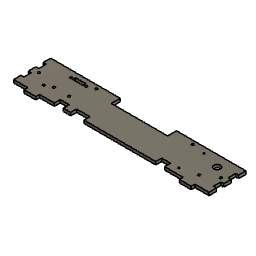
move_base_sidewall_1 (Autodesk Fusion 360 design; units mm, degrees)
Autodesk Fusion 360 part; units mm, degrees
note: some values were not read from the file. Set by a fixed rule: which sketch regions a step uses.
sketch "スケッチ1" plane through (0, 0, 0) normal (0, 1, 0) x (1, 0, 0)
  line L0 (-132, 0) -> (132, 0)
  line L1 (-132, 0) -> (-132, -10)
  line L2 (-132, -10) -> (-128, -10)
  line L3 (-128, -10) -> (-128, -20)
  line L4 (-128, -20) -> (-132, -20)
  line L5 (-132, -20) -> (-132, -30)
  line L6 (-132, -30) -> (-128, -30)
  line L7 (-128, -30) -> (-128, -40)
  line L8 (-128, -40) -> (-132, -40)
  line L9 (-132, -40) -> (-132, -50)
  line L10 (-132, -50) -> (-77, -50)
  line L11 (-77, -50) -> (-77, -42)
  line L12 (132, 0) -> (132, -10)
  line L13 (132, -10) -> (128, -10)
  line L14 (128, -10) -> (128, -20)
  line L15 (128, -20) -> (132, -20)
  line L16 (132, -20) -> (132, -30)
  line L17 (132, -30) -> (128, -30)
  line L18 (128, -30) -> (128, -40)
  line L19 (128, -40) -> (132, -40)
  line L20 (132, -40) -> (132, -50)
  line L21 (132, -50) -> (72, -50)
  line L22 (72, -50) -> (72, -42)
  line L23 (-77, -42) -> (-65, -42)
  line L24 (-65, -42) -> (-65, -50)
  line L25 (-37, -50) -> (60, -50)
  line L26 (60, -50) -> (60, -42)
  line L27 (60, -42) -> (72, -42)
  line L28 (-113, -50) -> (-97, -50)
  line L29 (-97, -50) -> (-97, -55)
  line L30 (-97, -55) -> (-113, -55)
  line L31 (-113, -55) -> (-113, -50)
  line L32 (97, -50) -> (113, -50)
  line L33 (113, -50) -> (113, -55)
  line L34 (113, -55) -> (97, -55)
  line L35 (97, -55) -> (97, -50)
  line L36 (-38, 0) -> (38, 0)
  line L37 (38, 0) -> (38, -12)
  line L38 (38, -12) -> (-38, -12)
  line L39 (-38, -12) -> (-38, 0)
  line L40 (-37, -50) -> (-37, -42)
  line L41 (-37, -42) -> (-55, -42)
  line L42 (-55, -42) -> (-55, -50)
  line L43 (-55, -50) -> (-65, -50)
  point P0 (0, -20)
  point P1 (-105, -50)
  point P2 (105, -50)
  dimension "d1" = 264
  dimension "d2" = 10
  dimension "d3" = 10
  dimension "d4" = 10
  dimension "d5" = 10
  dimension "d6" = 10
  dimension "d7" = 4
  dimension "d8" = 55
  dimension "d9" = 4
  dimension "d10" = 60
  dimension "d11" = 8
  dimension "d28" = 12
  dimension "d40" = 16
  dimension "d41" = 5
  dimension "d42" = 105
  dimension "d43" = 105
  dimension "d48" = 12
  dimension "d62" = 12
  dimension "d63" = 76
  dimension "d64" = 10
  dimension "d65" = 18
  constraint horizontal L0
  constraint midpoint origin L0
  constraint perpendicular L0 L1
  constraint perpendicular L1 L2
  constraint perpendicular L0 L3
  constraint perpendicular L3 L4
  constraint perpendicular L4 L5
  constraint perpendicular L3 L6
  constraint perpendicular L6 L7
  constraint perpendicular L7 L8
  constraint perpendicular L8 L9
  constraint perpendicular L9 L10
  constraint perpendicular L10 L11
  constraint collinear L1 L5
  constraint collinear L5 L9
  constraint collinear L3 L7
  constraint perpendicular L0 L12
  constraint perpendicular L12 L13
  constraint perpendicular L0 L14
  constraint perpendicular L14 L15
  constraint perpendicular L15 L16
  constraint perpendicular L14 L17
  constraint perpendicular L15 L18
  constraint perpendicular L14 L19
  constraint perpendicular L19 L20
  constraint perpendicular L14 L21
  constraint perpendicular L19 L22
  constraint collinear L12 L16
  constraint collinear L16 L20
  constraint collinear L14 L18
  constraint collinear L2 L13
  constraint collinear L4 L15
  constraint collinear L6 L17
  constraint collinear L8 L19
  constraint collinear L10 L21
  constraint perpendicular L11 L23
  constraint perpendicular L23 L24
  constraint vertical origin P0
  constraint collinear L23 L27
  constraint horizontal L28
  constraint vertical L29
  constraint horizontal L30
  constraint vertical L31
  constraint horizontal L32
  constraint vertical L33
  constraint horizontal L34
  constraint vertical L35
  constraint midpoint L28 P1
  constraint midpoint L32 P2
  constraint coincident L10 P1
  constraint coincident L21 P2
  constraint equal L29 L35
  constraint equal L30 L34
  constraint horizontal L25
  constraint collinear L21 L25
  constraint perpendicular L25 L26
  constraint horizontal L36
  constraint vertical L37
  constraint horizontal L38
  constraint vertical L39
  constraint midpoint origin L36
  constraint perpendicular L25 L40
  constraint perpendicular L40 L41
  constraint perpendicular L41 L42
  constraint perpendicular L24 L43
  constraint collinear L25 L43
  constraint collinear L23 L41
  measures "d1" distance of L0.start L0.end
  measures "d2" distance of L0.start L1.end
  measures "d3" distance of L2.end L3.end
  measures "d4" distance of L4.end L5.end
  measures "d5" distance of L6.end L7.end
  measures "d6" distance of L8.end L9.end
  measures "d7" distance of L1.end L2.end
  measures "d8" distance of L9.end L10.end
  measures "d9" distance of L12.end L13.end
  measures "d10" distance of L20.end L21.end
  measures "d11" distance of L21.end L22.end
  measures "d28" distance of L22.end L26.end
  measures "d40" distance of L29.end L30.end
  measures "d41" distance of L28.start L30.end
  measures "d42" horizontal distance of origin P1
  measures "d43" horizontal distance of origin P2
  measures "d48" distance of L11.end L23.end
  measures "d62" distance of L36.start L38.end
  measures "d63" distance of L37.end L38.end
  measures "d64" distance of L24.end L42.end
  measures "d65" distance of L40.end L41.end
extrude "押し出し1" add sketch "スケッチ1" along normal blind 4 contours L0 L1 L2 L3 L4 L5 L6 L7 L8 L9 L10 L11 L12 L13 L14 L15 L16 L17 L18 L19 L20 L21 L22 L23 L24 L25 L26 L27 L28 L32 L37 L38 L39 L40 L41 L42 L43 | L10 L28 L29 L30 L31 | L21 L32 L33 L34 L35
sketch "スケッチ2" plane through (0, 4, 0) normal (0, 1, 0) x (-1, 0, 0)
  line L0 (-72, 42) -> (-72, 50)
  line L1 (-72, 50) -> (-97, 50)
  line L2 (-132, 50) -> (-132, 40)
  line L3 (-132, 40) -> (-128, 40)
  line L4 (-128, 40) -> (-128, 30)
  line L5 (-128, 30) -> (-132, 30)
  line L6 (-132, 30) -> (-132, 20)
  line L7 (-132, 20) -> (-128, 20)
  line L8 (-128, 20) -> (-128, 10)
  line L9 (-128, 10) -> (-132, 10)
  line L10 (-132, 10) -> (-132, 0)
  line L11 (38, 0) -> (132, 0)
  line L12 (65, 5) -> (-65, 5)
  line L13 (123, 25) -> (-123, 25)
  line L14 (105, 36.5) -> (-105, 36.5)
  line L15 (37, 50) -> (-60, 50)
  line L16 (-60, 50) -> (-60, 42)
  line L17 (-60, 42) -> (-72, 42)
  line L18 (132, 0) -> (132, 10)
  line L19 (132, 10) -> (128, 10)
  line L20 (128, 10) -> (128, 20)
  line L21 (128, 20) -> (132, 20)
  line L22 (132, 20) -> (132, 30)
  line L23 (132, 30) -> (128, 30)
  line L24 (128, 30) -> (128, 40)
  line L25 (128, 40) -> (132, 40)
  line L26 (132, 40) -> (132, 50)
  line L27 (132, 50) -> (113, 50)
  line L28 (77, 50) -> (77, 42)
  line L29 (77, 42) -> (65, 42)
  line L30 (65, 42) -> (65, 50)
  line L31 (113, 50) -> (113, 55)
  line L32 (113, 55) -> (97, 55)
  line L33 (97, 55) -> (97, 50)
  line L34 (97, 50) -> (77, 50)
  line L35 (-97, 50) -> (-97, 55)
  line L36 (-97, 55) -> (-113, 55)
  line L37 (-113, 55) -> (-113, 50)
  line L38 (-113, 50) -> (-132, 50)
  line L39 (-38, 0) -> (-38, 12)
  line L40 (-38, 12) -> (38, 12)
  line L41 (38, 12) -> (38, 0)
  line L42 (-132, 0) -> (-38, 0)
  line L43 (65, 50) -> (55, 50)
  line L44 (55, 50) -> (55, 42)
  line L45 (55, 42) -> (37, 42)
  line L46 (37, 42) -> (37, 50)
  dimension "d14" = 5
  dimension "d15" = 65
  dimension "d16" = 65
  dimension "d17" = 25
  dimension "d19" = 5
  dimension "d24" = 105
  dimension "d25" = 105
  dimension "d46" = 13.5
  dimension "d47" = 5
  constraint parallel L11 L12
  constraint horizontal L13
  constraint horizontal L14
  measures "d14" distance of L11 L12
  measures "d15" horizontal distance of origin L12.start
  measures "d16" horizontal distance of origin L12.end
  measures "d17" distance of origin L13
  measures "d19" distance of L8 L13.end
  measures "d24" horizontal distance of origin L14.start
  measures "d25" horizontal distance of origin L14.end
  measures "d46" distance of L1 L14
  measures "d47" distance of L13.start L20
hole "穴1" at (-65, 4, 5) at (-123, 4, 25) at (65, 4, 5) at (123, 4, 25) at (-105, 4, 36.5) at (105, 4, 36.5) direction (0, -1, 0) diameter 3.2 end through all
sketch "スケッチ3" plane through (0, 4, 0) normal (0, 1, 0) x (-1, 0, 0)
  circle A0 centre (-65, 5) radius 1.6
  circle A1 centre (123, 25) radius 1.6
  circle A2 centre (-123, 25) radius 1.6
  circle A3 centre (-105, 36.5) radius 1.6
  line L0 (132, 0) -> (132, 10)
  line L1 (132, 10) -> (128, 10)
  line L2 (128, 10) -> (128, 20)
  line L3 (128, 20) -> (132, 20)
  line L4 (132, 20) -> (132, 30)
  line L5 (132, 30) -> (128, 30)
  line L6 (128, 30) -> (128, 40)
  line L7 (128, 40) -> (132, 40)
  line L8 (132, 40) -> (132, 50)
  line L9 (132, 50) -> (113, 50)
  line L10 (77, 50) -> (77, 42)
  line L11 (77, 42) -> (65, 42)
  line L12 (65, 42) -> (65, 50)
  line L13 (37, 50) -> (-60, 50)
  line L14 (-60, 50) -> (-60, 42)
  line L15 (-60, 42) -> (-72, 42)
  line L16 (-72, 42) -> (-72, 50)
  line L17 (-72, 50) -> (-97, 50)
  line L18 (-132, 50) -> (-132, 40)
  line L19 (-132, 40) -> (-128, 40)
  line L20 (-128, 40) -> (-128, 30)
  line L21 (-128, 30) -> (-132, 30)
  line L22 (-132, 30) -> (-132, 20)
  line L23 (-132, 20) -> (-128, 20)
  line L24 (-128, 20) -> (-128, 10)
  line L25 (-128, 10) -> (-132, 10)
  line L26 (-132, 10) -> (-132, 0)
  line L27 (38, 0) -> (132, 0)
  circle A4 centre (-108, 15) radius 4.5
  circle A5 centre (-83, 25) radius 15
  line L28 (-83, 8) -> (-83, 42)
  line L29 (113, 50) -> (113, 55)
  line L30 (113, 55) -> (97, 55)
  line L31 (97, 55) -> (97, 50)
  line L32 (97, 50) -> (77, 50)
  line L33 (-97, 50) -> (-97, 55)
  line L34 (-97, 55) -> (-113, 55)
  line L35 (-113, 55) -> (-113, 50)
  line L36 (-113, 50) -> (-132, 50)
  line L37 (75, 9) -> (95.5, 9)
  line L38 (95.5, 9) -> (95.5, 32)
  line L39 (95.5, 32) -> (75, 32)
  line L40 (75, 32) -> (75, 9)
  line L41 (75, 9) -> (95.5, 32) construction
  line L42 (95.5, 9) -> (75, 32) construction
  line L43 (78.25, 6.1) -> (92.25, 6.1)
  line L44 (92.25, 6.1) -> (92.25, 10.1)
  line L45 (92.25, 10.1) -> (78.25, 10.1)
  line L46 (78.25, 10.1) -> (78.25, 6.1)
  line L47 (78.25, 6.1) -> (92.25, 10.1) construction
  line L48 (92.25, 6.1) -> (78.25, 10.1) construction
  line L49 (-38, 0) -> (-38, 12)
  line L50 (-38, 12) -> (38, 12)
  line L51 (38, 12) -> (38, 0)
  line L52 (-132, 0) -> (-38, 0)
  line L53 (65, 50) -> (55, 50)
  line L54 (55, 50) -> (55, 42)
  line L55 (55, 42) -> (37, 42)
  line L56 (37, 42) -> (37, 50)
  point P0 (85.25, 20.5)
  point P1 (85.25, 8.1)
  dimension "d29" = 34
  dimension "d30" = 30
  dimension "d31" = 9
  dimension "d32" = 15
  dimension "d33" = 20
  dimension "d34" = 25
  dimension "d35" = 45
  dimension "d51" = 23
  dimension "d52" = 20.5
  dimension "d53" = 4
  dimension "d54" = 14
  dimension "d55" = 12.4
  dimension "d56" = 75
  dimension "d57" = 9
  constraint vertical L28
  constraint midpoint A5.centre L28
  constraint horizontal L37
  constraint perpendicular L37 L38
  constraint parallel L37 L39
  constraint parallel L38 L40
  constraint coincident L41 P0
  constraint coincident L42 P0
  constraint horizontal L43
  constraint perpendicular L43 L44
  constraint parallel L43 L45
  constraint parallel L44 L46
  constraint coincident L47 P1
  constraint coincident L48 P1
  constraint vertical P0 P1
  measures "d29" distance of L28.start L28.end
  measures "d30" diameter of A5
  measures "d31" diameter of A4
  measures "d32" distance of L27 A4.centre
  measures "d33" distance of L24 A4.centre
  measures "d34" distance of L27 A5.centre
  measures "d35" distance of L24 A5.centre
  measures "d51" distance of L37.start L39.end
  measures "d52" distance of L38.end L39.end
  measures "d53" distance of L43.start L45.end
  measures "d54" distance of L43.start L43.end
  measures "d55" distance of P0 P1
  measures "d56" distance of origin L40
  measures "d57" distance of origin L37
extrude "押し出し2" cut sketch "スケッチ3" against normal through all contours A4
hole "穴2" at (83, 4, 42) at (83, 4, 8) direction (0, -1, 0) diameter 2.3 depth 35 tip angle 118
extrude "押し出し3" cut sketch "スケッチ3" against normal through all contours L37 L44 L45 L46 | L37 L43 L44 L46
hole "穴3" at (-95.5, 4, 9) at (-75, 4, 9) at (-75, 4, 32) at (-95.5, 4, 32) direction (0, -1, 0) diameter 3.2 depth 16 tip angle 118
